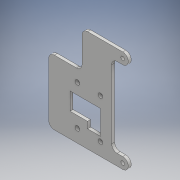
# Autodesk Inventor part: freestanding_cam_mount
Saved by Autodesk Inventor 2017 (Build 210142000, 142)
## iProperties
Created: 2018-01-26
Part Number: freestanding_cam_mount
Material: Generic
Document SubType Name: Modeling
Designer: Nic
Density: 1 g/cm^3
Appearance: Default
Author: Nic
Autodesk Inventor part; units mm, degrees
ref_plane "YZ Plane" through (0, 0, 0) normal (1, 0, 0) x (0, 1, 0)
ref_plane "XZ Plane" through (0, 0, 0) normal (0, 1, 0) x (-1, 0, 0)
ref_plane "XY Plane" through (0, 0, 0) normal (0, 0, 1) x (1, 0, 0)
sketch "Sketch1" plane through (0, 0, 0) normal (0, 1, 0) x (-1, 0, 0)
  circle A0 centre (0, 0) radius 1
  circle A1 centre (0, -49) radius 1
  arc A2 (0, 3) -> (0, -3) centre (0, 0) ccw
  arc A3 (0, -46) -> (0, -52) centre (0, -49) ccw
  line L0 (0, 3) -> (19, 3)
  line L1 (22, 0) -> (22, -14)
  line L2 (25, -17) -> (37, -17)
  line L3 (40, -20) -> (40, -49)
  line L4 (37, -52) -> (0, -52)
  line L5 (0, -3) -> (3, -3)
  line L6 (6, -6) -> (6, -43)
  line L7 (3, -46) -> (0, -46)
  arc A4 (6, -6) -> (3, -3) centre (3, -6) ccw
  arc A5 (22, 0) -> (19, 3) centre (19, 0) ccw
  arc A6 (22, -14) -> (25, -17) centre (25, -14) ccw
  arc A7 (40, -20) -> (37, -17) centre (37, -20) ccw
  arc A8 (37, -52) -> (40, -49) centre (37, -49) ccw
  arc A9 (3, -46) -> (6, -43) centre (3, -43) ccw
  circle A10 centre (12, -23.5) radius 1.25
  circle A11 centre (12, -45) radius 1.25
  circle A12 centre (24.5, -45) radius 1.25
  circle A13 centre (24.5, -23.5) radius 1.25
  line L8 (28.5, -29.5) -> (12, -29.5)
  line L9 (12, -29.5) -> (12, -42.5)
  line L10 (12, -42.5) -> (19, -42.5)
  line L11 (19, -42.5) -> (19, -39)
  line L12 (19, -39) -> (28.5, -39)
  line L13 (28.5, -39) -> (28.5, -29.5)
  line L14 (28.5, -34.25) -> (12, -34.25) construction
  point P0 (22, 3)
  point P1 (22, -17)
  point P2 (40, -52)
  dimension "d0" = 49
  dimension "d1" = 2
  dimension "d2" = 6
  dimension "d3" = 22
  dimension "d4" = 20
  dimension "d5" = 40
  dimension "d6" = 6
  dimension "d7" = 3
  dimension "d14" = 2.5
  dimension "d15" = 12.5
  dimension "d16" = 12
  dimension "d17" = 9.5
  dimension "d18" = 3.5
  dimension "d19" = 7
  dimension "d20" = 21.5
  dimension "d21" = 7
  constraints: 30 end point, 16 point on circle, 16 tangent, 14 centre point, 12 perpendicular, 9 equal radius, 7 point on line, 4 horizontal, 4 vertical alignment, 3 coincident, 2 horizontal alignment, 1 midpoint, 1 other
  measures "d0" distance of A1.centre point (0, 0)
  measures "d1" diameter of A0
  measures "d2" diameter of A2
  measures "d3" distance of L0.start point (22, 3)
  measures "d4" distance of point (22, 3) point (22, -17)
  measures "d5" distance of point (40, -52) L4.end
  measures "d6" distance from line of L6 point (0, 0)
  measures "d7" radius of A4
  measures "d14" diameter of A11
  measures "d15" distance of A11.centre A12.centre
  measures "d16" distance from line of A3.centre L9
  measures "d17" distance of L11.end L12.end
  measures "d18" distance of L10.end L11.end
  measures "d19" distance of L9.end L10.end
  measures "d20" distance of A12.centre A13.centre
  measures "d21" distance from line of L4 A12.centre
extrude "Extrusion1" add sketch "Sketch1" along normal blind 1.615
body "Solid1"
